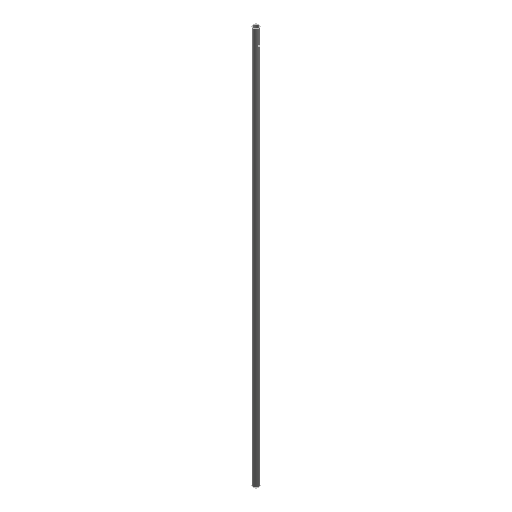
# Autodesk Inventor part: COTS_CarbonCenter_Fiberglass_30x28x2000mm_Pipe
Saved by Autodesk Inventor 2026 (Build 300175000, 175)
## iProperties
Created: 2025-06-20
Part Number: COTS_CarbonCenter_Fiberglass_30x28x2000mm_Pipe
Material: Generic
Document SubType Name: Modeling
Designer: User
Density: 1 g/cm^3
Appearance: Smooth - Black
Author: User
Autodesk Inventor part; units mm, degrees
ref_plane "YZ Plane" through (0, 0, 0) normal (1, 0, 0) x (0, 1, 0)
ref_plane "XZ Plane" through (0, 0, 0) normal (0, 1, 0) x (-1, 0, 0)
ref_plane "XY Plane" through (0, 0, 0) normal (0, 0, 1) x (1, 0, 0)
sketch "Sketch1" plane through (0, 0, 0) normal (0, 1, 0) x (-1, 0, 0)
  circle A0 centre (0, 0) radius 15
  circle A1 centre (0, 0) radius 14
  dimension "d0" = 30
  dimension "d1" = 28
  constraints: 2 centre point, 2 coincident
  measures "d0" diameter of A0
  measures "d1" diameter of A1
extrude "Extrusion1" add sketch "Sketch1" along normal blind 2000
sketch "Sketch2" plane through (0, 0, 0) normal (1, 0, 0) x (0, 1, 0)
  line L0 (2000, 14) -> (2000, -14) projected
  point P0 (0, 0)
  point P1 (1922, 0)
  dimension "d4" = 78
  constraints: 1 horizontal alignment
  measures "d4" distance from line of L0 point (1922, 0)
hole "Hole1" at (0, 1922, 0) direction (-1, 0, 0) diameter 5 end through all both
body "Solid1"
